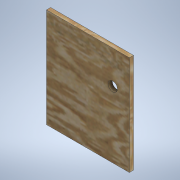
# Autodesk Inventor part: Shaft Mount
Saved by Autodesk Inventor 2020 (Build 240168000, 168)
## iProperties
Created: 2020-01-25
Part Number: Shaft Mount
Material: Wood (Maple)
Document SubType Name: Modeling
Designer: 1cikaychapman
Density: 0.67 g/cm^3
Appearance: Plywood - Weathered
Author: 1cikaychapman
Autodesk Inventor part; units mm, degrees
ref_plane "YZ Plane" through (0, 0, 0) normal (1, 0, 0) x (0, 1, 0)
ref_plane "XZ Plane" through (0, 0, 0) normal (0, 1, 0) x (-1, 0, 0)
ref_plane "XY Plane" through (0, 0, 0) normal (0, 0, 1) x (1, 0, 0)
sketch "Sketch1" plane through (0, 0, 0) normal (0, 0, 1) x (1, 0, 0)
  line L0 (0, 0) -> (254, 0)
  line L1 (254, 0) -> (254, 304.8)
  line L2 (254, 304.8) -> (0, 304.8)
  line L3 (0, 304.8) -> (0, 0)
  dimension "d0" = 254
  dimension "d1" = 304.8
  constraints: 8 end point, 2 parallel, 1 horizontal, 1 perpendicular
  measures "d0" distance of L1.end L2.end
  measures "d1" distance of L0.end L1.end
extrude "Extrusion1" add sketch "Sketch1" along normal blind 12.7
sketch "Sketch2" plane through (0, 0, 12.7) normal (0, 0, 1) x (1, 0, 0)
  line L0 (0, 0) -> (254, 0) projected
  line L1 (254, 0) -> (254, 304.8) projected
  point P0 (203.2, 203.2)
  dimension "d11" = 203.2
  dimension "d12" = 50.8
  measures "d11" distance from line of L0 point (203.2, 203.2)
  measures "d12" distance from line of L1 point (203.2, 203.2)
hole "Hole1" at (203.2, 203.2, 12.7) direction (0, 0, -1) diameter 28.575 end through all
body "Solid1"
